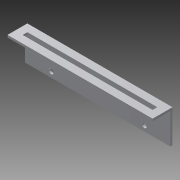
# Autodesk Inventor part: Fork 2 ver2
Saved by Autodesk Inventor 2015 (Build 190159000, 159)
## iProperties
Created: 2015-06-22
Part Number: Fork 2 ver2
Material: アルミニウム 5052 H32
Document SubType Name: シート メタル
Designer: kenta
Density: 2.68 g/cm^3
Sheet Metal Rule: Default_mm
Appearance: サテン
Author: kenta
Autodesk Inventor part; units mm, degrees
ref_plane "YZ Plane" through (0, 0, 0) normal (1, 0, 0) x (0, 1, 0)
ref_plane "XZ Plane" through (0, 0, 0) normal (0, 1, 0) x (-1, 0, 0)
ref_plane "XY Plane" through (0, 0, 0) normal (0, 0, 1) x (1, 0, 0)
sketch "スケッチ1" plane through (0, 0, 0) normal (0, 0, 1) x (1, 0, 0)
  line L0 (-47.5, 5.75) -> (47.5, 5.75)
  line L1 (47.5, 5.75) -> (47.5, -5.75)
  line L2 (47.5, -5.75) -> (-47.5, -5.75)
  line L3 (-47.5, -5.75) -> (-47.5, 5.75)
  line L4 (-47.5, 5.75) -> (47.5, -5.75) construction
  line L5 (47.5, 5.75) -> (-47.5, -5.75) construction
  point P0 (0, 0)
  dimension "d0" = 11.5
  dimension "d1" = 95
  constraints: 12 end point, 2 midpoint, 2 parallel, 1 horizontal, 1 perpendicular
  measures "d0" distance of L0.end L1.end
  measures "d1" distance of L1.end L2.end
extrude "押し出し1" add sketch "スケッチ1" along normal blind 1.5
sketch "スケッチ2" plane through (0, 0, 1.5) normal (0, 0, 1) x (1, 0, 0)
  line L0 (-42.5, 2.3) -> (42.5, 2.3)
  line L1 (42.5, 2.3) -> (42.5, -0.8)
  line L2 (42.5, -0.8) -> (-42.5, -0.8)
  line L3 (-42.5, -0.8) -> (-42.5, 2.3)
  line L4 (-47.5, -5.75) -> (47.5, -5.75) projected
  line L5 (47.5, -5.75) -> (47.5, 5.75) projected
  point P0 (0, 0)
  dimension "d8" = 3.1
  dimension "d9" = 85
  dimension "d10" = 4.95
  dimension "d11" = 5
  constraints: 8 end point, 2 parallel, 1 horizontal, 1 perpendicular
  measures "d8" distance of L0.end L1.end
  measures "d9" distance of L1.end L2.end
  measures "d10" distance between parallel lines of L4 L2
  measures "d11" distance between parallel lines of L1 L5
extrude "押し出し2" cut sketch "スケッチ2" against normal blind 1.5
sketch "スケッチ3" plane through (0, 0, 1.5) normal (0, 0, 1) x (1, 0, 0)
  line L0 (-47.5, 5.75) -> (47.5, 5.75)
  line L1 (47.5, 5.75) -> (47.5, 7.25)
  line L2 (47.5, 7.25) -> (-47.5, 7.25)
  line L3 (-47.5, 7.25) -> (-47.5, 5.75)
  point P0 (0, 0)
  dimension "d14" = 95
  dimension "d15" = 1.5
  constraints: 8 end point, 2 parallel, 1 horizontal, 1 perpendicular
  measures "d14" distance of L2.end L1.end
  measures "d15" distance of L1.end L0.end
extrude "押し出し3" add sketch "スケッチ3" against normal blind 21.5
sketch "スケッチ4" plane through (-47.5, 7.25, 1.5) normal (0, 1, 0) x (1, 0, 0)
  line L0 (95, 0) -> (0, 0) projected
  line L1 (0, 21.5) -> (95, 21.5) projected
  point P0 (47.5, 1.5)
  point P1 (17, 10)
  point P2 (78, 10)
  point P3 (17, 18)
  point P4 (78, 18)
  dimension "d18" = 30.5
  dimension "d19" = 30.5
  dimension "d21" = 8
  dimension "d29" = 3.5
  constraints: 2 horizontal alignment, 2 vertical alignment
  measures "d18" horizontal distance of point (17, 10) point (47.5, 1.5)
  measures "d19" horizontal distance of point (78, 10) point (47.5, 1.5)
  measures "d21" distance of point (17, 10) point (17, 18)
  measures "d29" distance from line of point (17, 18) L1
hole "穴1" at (-30.5, 7.25, -8.5) at (30.5, 7.25, -8.5) at (-30.5, 7.25, -16.5) at (30.5, 7.25, -16.5) direction (0, -1, 0) diameter 3.1 end through all
equation "\"d27\" = Thickness"
equation "\"BendRadius\" = Thickness"
equation "\"BendReliefWidth\" = Thickness"
equation "\"BendReliefDepth\" = 0.5 * Thickness"
equation "\"CornerReliefSize\" = 4 * Thickness"
equation "\"MinimumRemnant\" = 2 * Thickness"
equation "\"TransitionRadius\" = BendRadius"
equation "\"JacobiRadiusSize\" = BendRadius"
equation "\"GapSize\" = Thickness"
equation "\"Thickness\" = 0.5"
